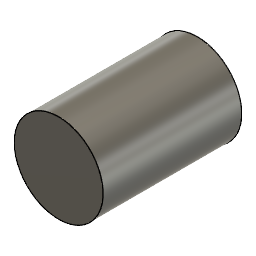
Pin (Autodesk Fusion 360 design; units mm, degrees)
part number: 2026-09-01-20-19-31-171
Autodesk Fusion 360 part; units mm, degrees
sketch "Sketch1" plane through (0, 0, 0) normal (0, 0, 1) x (1, 0, 0)
  circle A0 centre (0, 0) radius 6.25
sketch "Sketch2" plane through (0, 0, 0) normal (0, 0, 1) x (1, 0, 0)
  circle A0 centre (0, 0) radius 6.7276
extrude "Extrude2" add sketch "Sketch2" along normal blind 21
named bodies: "Pin_A500"
